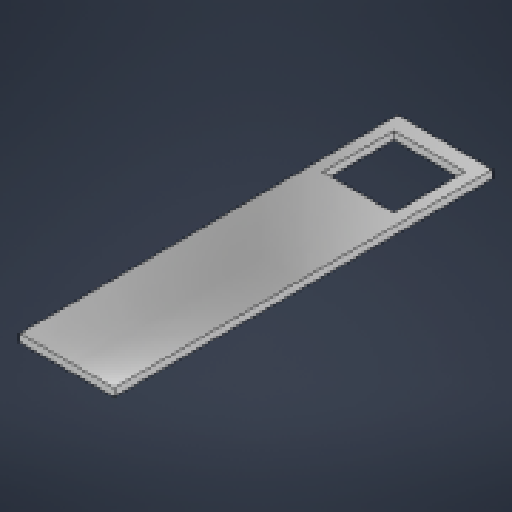
# Autodesk Inventor part: PLATE,FRONT
Saved by Autodesk Inventor 2026.1 (Build 301233020, 233B)
## iProperties
Created: 2026-03-19
Part Number: PLATE,FRONT
Material: Aluminum 6061
Document SubType Name: Sheet Metal
Designer: Owen L
Mass: 194.307 g
Surface Area: 373.864 cm^2
Volume: 71.9657 cm^3
Density: 2.7 g/cm^3
Sheet Metal Rule: Default
Appearance: Aluminum - Flat
Author: Owen L
Autodesk Inventor part; units mm, degrees
ref_plane "YZ Plane" through (0, 0, 0) normal (1, 0, 0) x (0, 1, 0)
ref_plane "XZ Plane" through (0, 0, 0) normal (0, 1, 0) x (-1, 0, 0)
ref_plane "XY Plane" through (0, 0, 0) normal (0, 0, 1) x (1, 0, 0)
sketch "Sketch1" plane through (0, 0, 0) normal (0, 1, 0) x (-1, 0, 0)
  line L0 (-31.75, -177.8) -> (31.75, -177.8)
  line L1 (31.75, -177.8) -> (31.75, 177.8)
  line L2 (31.75, 177.8) -> (-31.75, 177.8)
  line L3 (-31.75, 177.8) -> (-31.75, -177.8)
  line L4 (-31.75, -177.8) -> (31.75, 177.8) construction
  line L5 (31.75, -177.8) -> (-31.75, 177.8) construction
  line L6 (15.875, -152.4) -> (-15.875, -152.4)
  line L7 (-15.875, -152.4) -> (-15.875, -95.25)
  line L8 (-15.875, -95.25) -> (15.875, -95.25)
  line L9 (15.875, -95.25) -> (15.875, -152.4)
  line L10 (-15.875, 171.45) -> (15.875, 171.45)
  line L11 (15.875, 171.45) -> (15.875, 114.3)
  line L12 (15.875, 114.3) -> (-15.875, 114.3)
  line L13 (-15.875, 114.3) -> (-15.875, 171.45)
  point P0 (0, 0)
  point P1 (0, -95.25)
  point P2 (0, 114.3)
  dimension "d0" = 31.75
  dimension "d1" = 57.15
  dimension "d2" = 355.6
  dimension "d3" = 25.4
  dimension "d4" = 63.5
  dimension "d6" = 6.35
  measures "d0" distance of L7.end L8.end
  measures "d1" distance of L6.end L7.end
  measures "d2" distance of L2.end L0.start
  measures "d3" distance between parallel lines of L0 L6
  measures "d4" distance of L0.start L0.end
  measures "d6" distance between parallel lines of L2 L10
extrude "Plate1" add sketch "Sketch1" along normal blind 4.7625
sketch "Sketch2" plane through (0, 4.7625, 0) normal (0, 1, 0) x (1, 0, 0)
  circle A0 centre (0, -82.55) radius 25.4
  circle A1 centre (0, -25.4) radius 24.0284
  point P0 (0, 0)
  dimension "d7" = 50.8
  dimension "d8" = 82.55
  dimension "d9" = 48.0568
  dimension "d10" = 57.15
  constraints: 2 centre point, 2 vertical alignment
  measures "d7" diameter of A0
  measures "d8" distance of point (0, 0) A0.centre
  measures "d9" diameter of A1
  measures "d10" distance of A0.centre A1.centre
extrude "Cut1" cut sketch "Sketch2" against normal blind 4.7625
sketch "Sketch3" plane through (0, 4.7625, 0) normal (0, 1, 0) x (1, 0, 0)
  line L0 (31.75, 177.8) -> (31.75, -177.8) construction
  line L1 (31.75, -177.8) -> (-31.75, -177.8) construction
  circle A0 centre (0, -82.55) radius 25.4 projected
  point P0 (0, 0)
  point P1 (19.05, -107.95)
  point P2 (-19.05, -107.95)
  point P3 (19.05, -53.975)
  point P4 (-19.05, -53.975)
  point P5 (19.05, 0)
  point P6 (-19.05, 0)
  dimension "d13" = 12.7
  dimension "d16" = 38.1
  dimension "d19" = 53.975
  dimension "d22" = 28.575
  constraints: 1 horizontal, 1 vertical, 5 other
  measures "d13" distance from line of L0 point (19.05, -107.95)
  measures "d16" distance of point (19.05, -107.95) point (-19.05, -107.95)
  measures "d19" distance of point (19.05, -107.95) point (19.05, -53.975)
  measures "d22" vertical distance of A0.centre point (19.05, -53.975)
hole "Hole1" at (19.05, 4.7625, 107.95) at (-19.05, 4.7625, 107.95) at (19.05, 4.7625, 53.975) at (-19.05, 4.7625, 53.975) at (19.05, 4.7625, 0) at (-19.05, 4.7625, 0) direction (0, -1, 0) diameter 3.9624 end through all thread size "10-32 UNF" class "2B" standard "ANSI Unified Screw Threads"
equation "\"d11\" = Thickness"
equation "\"d28\" = Thickness"
equation "\"d5\" = Thickness"
equation "\"BendRadius\" = Thickness"
equation "\"BendReliefWidth\" = Thickness"
equation "\"BendReliefDepth\" = 0.5 * Thickness"
equation "\"CornerReliefSize\" = 4 * Thickness"
equation "\"MinimumRemnant\" = 2 * Thickness"
equation "\"TransitionRadius\" = BendRadius"
equation "\"JacobiRadiusSize\" = BendRadius"
equation "\"GapSize\" = Thickness"
equation "\"Thickness\" = 4.7625"
body "Solid1"
